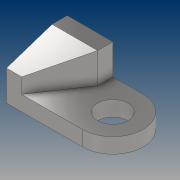
# Autodesk Inventor part: 27
Saved by Autodesk Inventor 2020.2 (Build 242310000, 310)
## iProperties
Created: 2020-09-17
Part Number: 27
Material: 鋼、碳鋼
Document SubType Name: Modeling
Designer: user
Density: 7.85 g/cm^3
Appearance: 半拋光
Mass: 303.337 g
Surface Area: 94.0824 cm^2
Volume: 38.6416 cm^3
Author: user
Autodesk Inventor part; units mm, degrees
ref_plane "YZ Plane" through (0, 0, 0) normal (1, 0, 0) x (0, 1, 0)
ref_plane "XZ Plane" through (0, 0, 0) normal (0, 1, 0) x (-1, 0, 0)
ref_plane "XY Plane" through (0, 0, 0) normal (0, 0, 1) x (1, 0, 0)
sketch "草圖1" plane through (0, 0, 0) normal (0, 1, 0) x (-1, 0, 0)
  circle A0 centre (0, 0) radius 20
  line L0 (0, -20) -> (50, -20)
  line L1 (50, -20) -> (50, 20)
  line L2 (50, 20) -> (0, 20)
  line L3 (0, 20) -> (0, -20)
  point P0 (0, 20)
  dimension "d0" = 40
  dimension "d1" = 50
  constraints: 8 end point, 3 horizontal, 2 parallel, 1 coincident, 1 perpendicular, 3 other
  measures "d1" distance of L0.start L0.end
extrude "擠出1" add sketch "草圖1" along normal blind 10
sketch "草圖2" plane through (0, 10, 0) normal (0, 1, 0) x (1, 0, 0)
  line L0 (-50, -20) -> (-50, 20) projected
  line L1 (-50, 20) -> (0, 20) projected
  arc A0 (0, -20) -> (0, 20) centre (0, 0) ccw projected
  line L2 (0, -20) -> (-50, -20) projected
  line L3 (-50, -20) -> (-50, 20) projected
  line L4 (-50, 20) -> (0, 20) projected
  arc A1 (0, -20) -> (0, 20) centre (0, 0) ccw projected
  line L5 (0, -20) -> (-50, -20) projected
  line L6 (0, 20) -> (-50, 20) projected
  line L7 (-50, 20) -> (-20, 20)
  line L8 (-20, 20) -> (-20, -20)
  line L9 (-20, -20) -> (-50, -20)
  line L10 (-50, -20) -> (-50, 20)
  line L11 (-50, -20) -> (0, -20) projected
  point P0 (-20, -20)
  point P1 (-20, 20)
  dimension "d4" = 30
  constraints: 8 end point, 2 parallel, 1 collinear, 1 horizontal, 1 perpendicular
  measures "d4" distance between parallel lines of L0 L8
extrude "擠出2" add sketch "草圖2" along normal blind 20 contours L0 L1 L8 L2
sketch "草圖3" plane through (0, 30, 0) normal (0, 1, 0) x (1, 0, 0)
  line L0 (-50, -20) -> (-50, 20) projected
  line L1 (-50, 20) -> (-20, 20) projected
  line L2 (-20, 20) -> (-20, -20) projected
  line L3 (-20, -20) -> (-50, -20) projected
  line L4 (-20, 10) -> (-40, -20)
  point P0 (0, 0)
  dimension "d7" = 10
  dimension "d8" = 10
  constraints: 2 end point, 2 point on line
  measures "d7" distance from line of L1 L4.start
  measures "d8" distance from line of L4.end L0
extrude "擠出3" cut sketch "草圖3" against normal up to surface (20 mm away) contours L4 L2 L3
sketch "草圖6" plane through (-20, 10, -20) normal (1, 0, 0) x (0, 0, -1)
  line L0 (-10, 0) -> (-10, 20) projected
  line L1 (-10, 20) -> (0, 20) projected
  line L2 (0, 20) -> (0, 0) projected
  line L3 (-10, 0) -> (0, 0) projected
  line L4 (-40, 0) -> (-10, 0) projected
  line L5 (-40, -10) -> (-40, 0) projected
  line L6 (0, -10) -> (-40, -10) projected
  line L7 (0, 0) -> (0, -10) projected
  line L8 (-10, 20) -> (-10, 0) projected
  line L9 (-10, 20) -> (-40, 10)
  line L10 (-40, 10) -> (-10, 10)
  line L11 (-10, 10) -> (-10, 20)
  line L12 (-40, 0) -> (-40, 20) projected
  line L13 (-40, 20) -> (-10, 20) projected
  point P0 (-20, -10)
  dimension "d14" = 10
  constraints: 6 end point, 2 midpoint, 2 perpendicular
  measures "d14" distance from line of L13 L9.end
extrude "擠出4" cut sketch "草圖6" against normal blind 85.25 contours L9 L12 L13
sketch "草圖7" plane through (0, 10, 0) normal (0, 1, 0) x (1, 0, 0)
  arc A0 (0, -20) -> (0, 20) centre (0, 0) ccw projected
  constraints: 1 coincident
hole "孔1" at (0, 10, 0) direction (0, -1, 0) diameter 20 end through all
